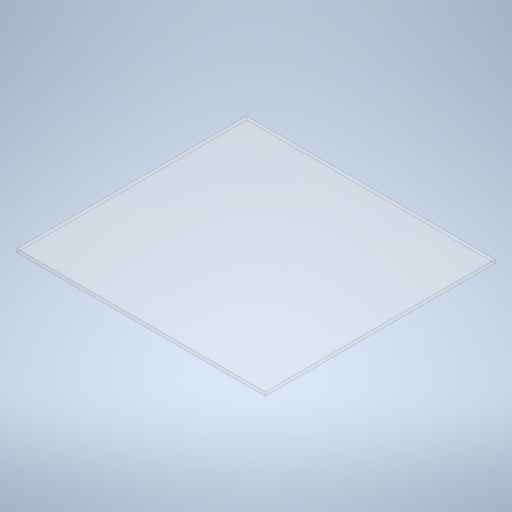
# Autodesk Inventor part: touch_panel
Saved by Autodesk Inventor 2023 (Build 270158000, 158)
## iProperties
Created: 2023-03-12
Part Number: touch_panel
Material: Glass
Document SubType Name: Modeling
Designer: nigel
Density: 2.18 g/cm^3
Appearance: Clear
Author: nigel
Autodesk Inventor part; units mm, degrees
ref_plane "YZ Plane" through (0, 0, 0) normal (1, 0, 0) x (0, 1, 0)
ref_plane "XZ Plane" through (0, 0, 0) normal (0, 1, 0) x (-1, 0, 0)
ref_plane "XY Plane" through (0, 0, 0) normal (0, 0, 1) x (1, 0, 0)
sketch "Sketch1" plane through (0, 0, 0) normal (0, 1, 0) x (-1, 0, 0)
  line L0 (16.75, 15.5) -> (-16.75, 15.5)
  line L1 (-16.75, 15.5) -> (-16.75, -15.5)
  line L2 (-16.75, -15.5) -> (16.75, -15.5)
  line L3 (16.75, -15.5) -> (16.75, 15.5)
  line L4 (16.75, 15.5) -> (-16.75, -15.5) construction
  line L5 (-16.75, 15.5) -> (16.75, -15.5) construction
  point P0 (0, 0)
  dimension "d0" = 31
  dimension "d1" = 33.5
  constraints: 12 end point, 2 midpoint, 2 parallel, 1 horizontal, 1 perpendicular
  measures "d0" distance of L2.end L0.start
  measures "d1" distance of L0.start L0.end
extrude "Extrusion1" add sketch "Sketch1" along normal blind 0.5
sketch "Sketch2" plane through (0, 0.5, 0) normal (0, 1, 0) x (1, 0, 0)
  line L0 (-16.75, -15.5) -> (16.75, -15.5) projected
  line L1 (-15.9661, -15.5) -> (-7.7382, -15.5)
  line L2 (-7.7382, -15.5) -> (-7.7382, -17.215)
  line L3 (-7.7382, -17.215) -> (-15.9661, -17.215)
  line L4 (-15.9661, -17.215) -> (-15.9661, -15.5)
  line L5 (-14.203, -17.215) -> (-9.5503, -17.215)
  line L6 (-9.5503, -17.215) -> (-9.5503, -18.8312)
  line L7 (-9.5503, -18.8312) -> (-14.203, -18.8312)
  line L8 (-14.203, -18.8312) -> (-14.203, -17.215)
  point P0 (0, 0)
  constraints: 16 end point, 4 parallel, 2 horizontal, 2 perpendicular, 2 point on line
body "Solid1"
